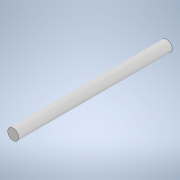
# Autodesk Inventor part: mouth_horizontal_rod
Saved by Autodesk Inventor 2021 (Build 250183000, 183)
## iProperties
Created: 2023-06-07
Part Number: mouth_horizontal_rod
Material: Generic
Document SubType Name: Modeling
Designer: LENOVO
Density: 1 g/cm^3
Appearance: Default
Author: LENOVO
Autodesk Inventor part; units mm, degrees
ref_plane "YZ Plane" through (0, 0, 0) normal (1, 0, 0) x (0, 1, 0)
ref_plane "XZ Plane" through (0, 0, 0) normal (0, 1, 0) x (-1, 0, 0)
ref_plane "XY Plane" through (0, 0, 0) normal (0, 0, 1) x (1, 0, 0)
sketch "Sketch1" plane through (0, 0, 0) normal (0, 0, 1) x (1, 0, 0)
  circle A0 centre (0, 0) radius 2.5
  dimension "d0" = 5
  constraints: 1 centre point, 1 coincident
  measures "d0" diameter of A0
extrude "Extrusion1" add sketch "Sketch1" along normal blind 70
body "Solid1"
